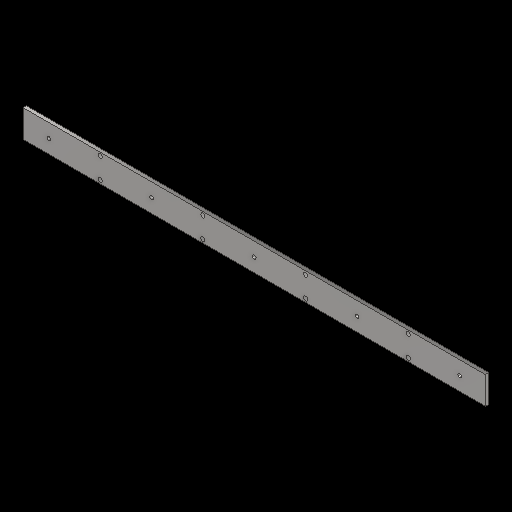
# Autodesk Inventor part: Rail_bracket
Saved by Autodesk Inventor 2026.1 (Build 301233000, 233)
## iProperties
Created: 2024-12-30
Part Number: Rail_bracket
Material: Stainless Steel
Document SubType Name: Modeling
Designer: drago
Density: 8 g/cm^3
Appearance: Semi-Polished
Author: drago
Autodesk Inventor part; units mm, degrees
ref_plane "YZ Plane" through (0, 0, 0) normal (1, 0, 0) x (0, 1, 0)
ref_plane "XZ Plane" through (0, 0, 0) normal (0, 1, 0) x (-1, 0, 0)
ref_plane "XY Plane" through (0, 0, 0) normal (0, 0, 1) x (1, 0, 0)
sketch "Sketch1" plane through (0, 0, 0) normal (0, 0, 1) x (1, 0, 0)
  line L0 (0, 0) -> (675, 0)
  line L1 (675, 0) -> (675, 40)
  line L2 (675, 40) -> (0, 40)
  line L3 (0, 40) -> (0, 0)
  line L4 (0, 20) -> (675, 20) construction
  line L5 (0, 5) -> (675, 5) construction
  line L6 (0, 35) -> (675, 35) construction
  line L7 (337.5, 40) -> (337.5, 0) construction
  circle A0 centre (37.5, 20) radius 2.6
  circle A1 centre (187.5, 20) radius 2.6
  circle A2 centre (337.5, 20) radius 2.6
  circle A3 centre (487.5, 20) radius 2.6
  circle A4 centre (637.5, 20) radius 2.6
  circle A5 centre (112.5, 5) radius 3
  circle A6 centre (262.5, 5) radius 3
  circle A7 centre (412.5, 5) radius 3
  circle A8 centre (562.5, 5) radius 3
  circle A9 centre (112.5, 35) radius 3
  circle A10 centre (262.5, 35) radius 3
  circle A11 centre (412.5, 35) radius 3
  circle A12 centre (562.5, 35) radius 3
  point P0 (37.5, 20)
  point P1 (112.5, 5)
  point P2 (262.5, 5)
  point P3 (412.5, 5)
  point P4 (562.5, 5)
  dimension "d16" = 675
  dimension "d17" = 40
  dimension "d20" = 37.5
  dimension "d22" = 5.2
  dimension "d25" = 150
  dimension "d31" = 75
  dimension "d32" = 6
  dimension "d35" = 150
  dimension "d42" = 150
  dimension "d47" = 30
  constraints: 16 end point, 14 coincident, 13 centre point, 7 point on line, 4 horizontal, 4 midpoint, 3 parallel, 1 equal radius, 1 perpendicular, 1 symmetric about line, 34 other
  measures "d16" distance of L2.end L1.end
  measures "d17" distance of L1.end L0.end
  measures "d20" distance from line of L3 point (37.5, 20)
  measures "d22" diameter of A0
  measures "d25" distance of A0.centre A1.centre
  measures "d31" horizontal distance of point (37.5, 20) point (112.5, 5)
  measures "d32" diameter of A5
  measures "d35" distance of A5.centre A6.centre
  measures "d42" distance of A9.centre A10.centre
  measures "d47" distance between parallel lines of L5 L6
extrude "Extrusion1" add sketch "Sketch1" against normal blind 5 contours L3 L2 L1 L0 | A0 | A1 | A2 | A3 | A4 | A5 | A6 | A7 | A8 | A9 | A10 | A11 | A12
hole "Hole1" at (37.5, 20, 0) at (187.5, 20, 0) at (337.5, 20, 0) at (487.5, 20, 0) at (637.5, 20, 0) direction (0, 0, -1) diameter 5.2 end through all
hole "Hole2" at (112.5, 5, 0) at (262.5, 5, 0) at (412.5, 5, 0) at (562.5, 5, 0) at (112.5, 35, 0) at (262.5, 35, 0) at (412.5, 35, 0) at (562.5, 35, 0) direction (0, 0, -1) diameter 6 end through all
thread "Thread9" size "M6x1" class "6H" standard "ISO Metric profile" full length
thread "Thread10" size "M6x1" class "6H" standard "ISO Metric profile" full length
thread "Thread11" size "M6x1" class "6H" standard "ISO Metric profile" full length
thread "Thread12" size "M6x1" class "6H" standard "ISO Metric profile" full length
thread "Thread13" size "M6x1" class "6H" standard "ISO Metric profile" full length
thread "Thread14" size "M6x1" class "6H" standard "ISO Metric profile" full length
thread "Thread15" size "M6x1" class "6H" standard "ISO Metric profile" full length
thread "Thread16" size "M6x1" class "6H" standard "ISO Metric profile" full length
body "Solid3"
